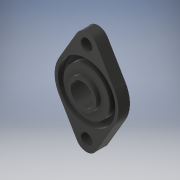
# Autodesk Inventor part: bearing
Saved by Autodesk Inventor 2019 (Build 230136000, 136)
## iProperties
Created: 2021-11-02
Part Number: bearing
Material: Generic
Document SubType Name: Modeling
Designer: modym
Density: 1 g/cm^3
Appearance: Smooth - Black
Author: modym
Autodesk Inventor part; units mm, degrees
ref_plane "YZ Plane" through (0, 0, 0) normal (1, 0, 0) x (0, 1, 0)
ref_plane "XZ Plane" through (0, 0, 0) normal (0, 1, 0) x (-1, 0, 0)
ref_plane "XY Plane" through (0, 0, 0) normal (0, 0, 1) x (1, 0, 0)
sketch "Sketch1" plane through (0, 0, 0) normal (0, 0, 1) x (1, 0, 0)
  circle A0 centre (0, 0) radius 10
  circle A1 centre (0, 35.5) radius 5
  circle A2 centre (0, -35.5) radius 5
  circle A3 centre (0, -35.5) radius 9.5
  circle A4 centre (0, 35.5) radius 9.5
  circle A5 centre (0, 0) radius 25
  circle A6 centre (0, 0) radius 20
  line L0 (-23.7028, 13.9437) -> (-8.1883, 40.3169)
  line L1 (8.1883, 40.3169) -> (23.7028, 13.9437)
  line L2 (8.1883, -40.3169) -> (23.7028, -13.9437)
  line L3 (-8.1883, -40.3169) -> (-23.7028, -13.9437)
  arc A7 (-4.4942, 27.1303) -> (-4.4942, -27.1303) centre (0, 0) ccw
  arc A8 (4.4942, -27.1303) -> (4.4942, 27.1303) centre (0, 0) ccw
  dimension "d0" = 20
  dimension "d4" = 10
  dimension "d5" = 10
  dimension "d7" = 19
  dimension "d8" = 50
  dimension "d9" = 40
  constraints: 16 point on circle, 9 centre point, 8 end point, 8 tangent, 6 coincident
  measures "d0" diameter of A0
  measures "d4" diameter of A1
  measures "d5" diameter of A2
  measures "d7" diameter of A4
  measures "d8" diameter of A5
  measures "d9" diameter of A6
extrude "Extrusion1" add sketch "Sketch1" along normal blind 10
sketch "Sketch2" plane through (0, 0, 10) normal (0, 0, 1) x (1, 0, 0)
  circle A0 centre (0, 0) radius 10
  circle A1 centre (0, 0) radius 12.5
  dimension "d14" = 25
  constraints: 2 centre point, 2 coincident
  measures "d14" diameter of A1
extrude "Extrusion2" add sketch "Sketch2" along normal blind 4
sketch "Sketch3" plane through (0, 0, 0) normal (0, 0, -1) x (-1, 0, 0)
  circle A0 centre (0, 0) radius 20
  circle A1 centre (0, 0) radius 25
  constraints: 2 centre point, 2 coincident
extrude "Extrusion3" add sketch "Sketch3" against normal blind 4
fillet "Fillet1" radius 2 1 edges at (-25, 0, 4)
body "Solid1"
